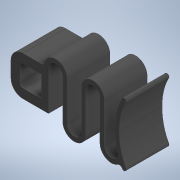
# Autodesk Inventor part: resortePlano1_2mmX3D
Saved by Autodesk Inventor 2021.5 (Build 255421000, 421)
## iProperties
Created: 2024-11-30
Part Number: resortePlano1_2mmX3D
Material: ABS NEGRO 4DLAB
Document SubType Name: Modeling
Designer: Joho_
Density: 0.894 g/cm^3
Appearance: Genérico(2)
Mass: 1.86881 g
Surface Area: 30.6443 cm^2
Volume: 2.09039 cm^3
Author: Joho_
## iProperties of the stored document _3DPrint.ipt
Created: 2024-11-30
Part Number: _3DPrint
Material: Genérico
Document SubType Name: Modeling
Designer: Joho_
Density: 1 g/cm^3
Appearance: Valor por defecto
Author: Joho_
Autodesk Inventor part; units mm, degrees
ref_plane "YZ Plane" through (0, 0, 0) normal (1, 0, 0) x (0, 1, 0)
ref_plane "XZ Plane" through (0, 0, 0) normal (0, 1, 0) x (-1, 0, 0)
ref_plane "XY Plane" through (0, 0, 0) normal (0, 0, 1) x (1, 0, 0)
sketch "Boceto1" plane through (0, 0, 0) normal (0, 0, 1) x (1, 0, 0)
  line L0 (3, -11.4) -> (3, -5.5)
  line L1 (3, -5.5) -> (-2.2, -5.5)
  arc A0 (-5.5, -2.2) -> (-2.2, -5.5) centre (-2.2, -2.2) ccw
  line L2 (-5.5, -2.2) -> (-5.5, 2.2)
  arc A1 (-2.2, 5.5) -> (-5.5, 2.2) centre (-2.2, 2.2) ccw
  line L3 (-2.2, 5.5) -> (3, 5.5)
  line L4 (3, 5.5) -> (3, 11.4)
  line L5 (3, 3) -> (-2.2, 3)
  arc A2 (-2.2, 3) -> (-3, 2.2) centre (-2.2, 2.2) ccw
  line L6 (-3, 2.2) -> (-3, -2.2)
  arc A3 (-3, -2.2) -> (-2.2, -3) centre (-2.2, -2.2) ccw
  line L7 (-2.2, -3) -> (3, -3)
  line L8 (3, -3) -> (3, 3)
  line L9 (-2.2, 3.25) -> (3.25, 3.25)
  line L10 (3.25, 3.25) -> (3.25, -3.25)
  line L11 (3.25, -3.25) -> (-2.2, -3.25)
  arc A4 (-3.25, -2.2) -> (-2.2, -3.25) centre (-2.2, -2.2) ccw
  line L12 (-3.25, -2.2) -> (-3.25, 2.2)
  arc A5 (-2.2, 3.25) -> (-3.25, 2.2) centre (-2.2, 2.2) ccw
  line L13 (-2.2, 5) -> (5, 5)
  line L14 (5, 5) -> (5, -5)
  line L15 (5, -5) -> (-2.2, -5)
  arc A6 (-5, -2.2) -> (-2.2, -5) centre (-2.2, -2.2) ccw
  line L16 (-5, -2.2) -> (-5, 2.2)
  arc A7 (-2.2, 5) -> (-5, 2.2) centre (-2.2, 2.2) ccw
  line L17 (23.6, 0) -> (22.4, 0)
  arc A8 (25.6, 8.5) -> (23.6, 0) centre (40.821, 0.4333) ccw
  circle A9 centre (23.6, 0) radius 1.2
  arc A10 (26.6603, 7.9381) -> (24.7996, 0.0302) centre (40.821, 0.4333) ccw
  line L18 (25.6, 8.5) -> (25.9736, 8.302)
  arc A11 (26.6603, 7.9381) -> (25.6, 8.5) centre (26.1301, 8.219) ccw
  arc A12 (23.6, 0) -> (25.6, -8.5) centre (40.821, -0.4333) ccw
  arc A13 (24.7996, -0.0302) -> (26.6603, -7.9381) centre (40.821, -0.4333) ccw
  line L19 (25.9736, -8.302) -> (26.6603, -7.9381)
  arc A14 (25.6, -8.5) -> (26.6603, -7.9381) centre (26.1301, -8.219) ccw
  line L20 (3, -5.5) -> (5, -5.5)
  line L21 (5, -5.5) -> (5, -5)
  line L22 (3, 5.5) -> (5, 5.5)
  line L23 (5, 5) -> (5, 5.5)
  line L24 (5, 5.5) -> (7, 5.5)
  line L25 (9, 5.5) -> (10.2, 5.5)
  line L26 (10.2, 5.5) -> (10.2, -5.5)
  line L27 (10.2, -5.5) -> (9, -5.5)
  line L28 (9, -5.5) -> (9, 5.5)
  line L29 (10.2, -5.5) -> (12.2, -5.5)
  arc A15 (10.2, 5.5) -> (3.8, 5.5) centre (7, 5.5) ccw
  arc A16 (9, 5.5) -> (5, 5.5) centre (7, 5.5) ccw
  line L30 (15.4, -5.5) -> (14.2, -5.5)
  line L31 (14.2, -5.5) -> (14.2, 5.5)
  line L32 (14.2, 5.5) -> (15.4, 5.5)
  line L33 (15.4, 5.5) -> (15.4, -5.5)
  arc A17 (10.2, -5.5) -> (14.2, -5.5) centre (12.2, -5.5) ccw
  arc A18 (9, -5.5) -> (15.4, -5.5) centre (12.2, -5.5) ccw
  line L34 (19.4, 5.5) -> (20.6, 5.5)
  line L35 (20.6, 5.5) -> (20.6, -5.5)
  line L36 (20.6, -5.5) -> (19.4, -5.5)
  line L37 (19.4, -5.5) -> (19.4, 5.5)
  line L38 (20.6, -5.5) -> (22.6, -5.5)
  arc A19 (20.6, 5.5) -> (14.2, 5.5) centre (17.4, 5.5) ccw
  arc A20 (19.4, 5.5) -> (15.4, 5.5) centre (17.4, 5.5) ccw
  arc A21 (20.6, -5.5) -> (24.5287, -6.0291) centre (22.6, -5.5) ccw
  arc A22 (19.4, -5.5) -> (25.1061, -7.4898) centre (22.6, -5.5) ccw
  point P0 (0, 0)
  point P1 (4.2, -5)
  point P2 (3.8, 5)
  point P3 (23, 0)
  point P4 (23.6116, -1.1999)
  point P5 (24.7996, 0.0302)
  point P6 (23.6116, 1.1999)
  dimension "d1" = 0.25
  dimension "d2" = 2
  dimension "d41" = 1.2
  dimension "d44" = 2
  dimension "d46" = 11
  dimension "d47" = 2
  dimension "d48" = 1.2
  dimension "d49" = 11
  dimension "d50" = 11
  dimension "d51" = 2
  constraints: 78 end point, 48 point on circle, 25 centre point, 8 horizontal, 6 coincident, 6 parallel, 4 perpendicular, 4 point on line, 1 collinear, 3 other
  measures "d1" distance between parallel lines of L5 L9
  measures "d2" distance between parallel lines of L5 L13
  measures "d41" radial gap between concentric circles of A8 A10
  measures "d44" distance of L22.end L24.end
  measures "d46" distance of L25.end L26.end
  measures "d47" distance of L26.end L29.end
  measures "d48" distance of L31.end L32.end
  measures "d49" distance of L30.end L31.end
  measures "d50" distance of L34.end L36.start
  measures "d51" distance of L36.start L38.end
extrude "Extrusión1" add sketch "Boceto1" along normal blind 12 contours L1 A0 L2 A1 L3 L22 L23 L13 A7 L16 A6 L15 L21 L20 | L15 A6 L16 A7 L13 L14 | L22 A15 L25 A16 | L25 L26 L27 L28 | L27 A17 L30 A18 | L30 L31 L32 L33 | L32 A19 L34 A20 | L34 L35 L36 L37 | L36 A21 A12 A22 | A12 A9 A13 A14 | A12 A8 A9 | A8 A11 A10 A9 | L9 L10 L11 A4 L12 A5
fillet "Empalme1" radius 0.8 3 edges at (3.8, 5.5, 6) (25.1061, -7.4898, 6) (24.5287, -6.0291, 6)
